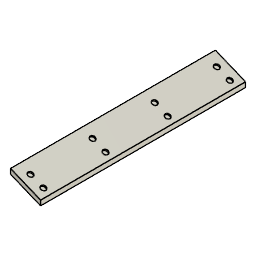
name_sign_LED_holder_bottom (Autodesk Fusion 360 design; units mm, degrees)
Autodesk Fusion 360 part; units mm, degrees
sketch "Name Sign LED Holder Bottom" plane through (0, 0, 0) normal (0, 1, 0) x (1, 0, 0)
  line L0 (-0.0003, -18.6907) -> (-0.0003, -13.2867)
  line L1 (32.3821, -5.4097) -> (32.3821, -0.0057)
  line L2 (-0.0003, -13.2867) -> (32.3821, -0.0057)
  line L3 (-0.0003, -18.6907) -> (32.3821, -5.4097)
  dimension "d36" = 5.404
  dimension "d37" = 5.404
  dimension "d38" = 112.3
  dimension "d39" = 35
  dimension "d40" = 4.9998
  constraint vertical L0
  constraint vertical L1
  measures "d36" distance of L0.start L0.end
  measures "d37" distance of L1.start L1.end
  measures "d38" angle of L0 L3
  measures "d39" distance of L0.end L1.end
  measures "d40" distance of L2 L3
extrude "Extrude1" add sketch "Name Sign LED Holder Bottom" along normal blind 220
sketch "Magnet Holes" plane through (6.5618, 0, 15.9994) normal (0.379456, 0, 0.92521) x (0, 1, 0)
  line L0 (0, 7.0925) -> (0, -27.9075)
  line L1 (0, -27.9075) -> (220, -27.9075)
  line L2 (220, -27.9075) -> (220, 7.0925)
  line L3 (220, 7.0925) -> (0, 7.0925)
  circle A0 centre (10, -20.4075) radius 2.75
  dimension "d50" = 5.5
  dimension "d51" = 10
  dimension "d52" = 7.5
  measures "d50" diameter of A0
  measures "d51" distance of L0 A0.centre
  measures "d52" distance of L1 A0.centre
extrude "Extrude4" cut sketch "Magnet Holes" against normal blind 1.5 contours A0
pattern_linear "R-Pattern1" count 4 spacing 66.6667 along (0, 1, 0) count 2 spacing 15 along (-0.92521, 0, 0.379456) of "Extrude4"
equation "d4 = 200 mm + 10 mm + 5 mm + 5 mm"
equation "magnet_hole_diameter = 5.5 mm"
equation "magnet_hole_depth = 1.5 mm"
equation "number_of_magnet_columns = 4"
equation "number_of_magnet_rows = 2"
equation "magnet_hole_side_offset = 10 mm"
equation "magnet_hole_top_offset = 7.5 mm"
equation "magnet_pattern_length = 220.00 mm - 2 * ( magnet_hole_side_offset )"
equation "magnet_pattern_height = 35.00 mm - vertical_part_width - 2 * ( magnet_hole_top_offset )"
equation "vertical_part_width = 5.00 mm"
equation "d50 = magnet_hole_diameter"
equation "d51 = magnet_hole_side_offset"
equation "d52 = magnet_hole_top_offset"
equation "d53 = -magnet_hole_depth"
equation "d55 = number_of_magnet_columns"
equation "d56 = number_of_magnet_rows"
equation "d57 = magnet_pattern_length"
equation "d58 = magnet_pattern_height"
named bodies: "Name Sign LED Holder Bottom"
